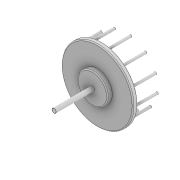
# Autodesk Inventor part: updated_base
Saved by Autodesk Inventor 2021 (Build 250183000, 183)
## iProperties
Created: 2021-06-23
Part Number: updated_base
Material: Generic
Document SubType Name: Modeling
Designer: Hp
Density: 1 g/cm^3
Appearance: Default
Mass: 195.945 g
Surface Area: 498.886 cm^2
Volume: 195.945 cm^3
Author: Hp
Autodesk Inventor part; units mm, degrees
ref_plane "YZ Plane" through (0, 0, 0) normal (1, 0, 0) x (0, 1, 0)
ref_plane "XZ Plane" through (0, 0, 0) normal (0, 1, 0) x (-1, 0, 0)
ref_plane "XY Plane" through (0, 0, 0) normal (0, 0, 1) x (1, 0, 0)
sketch "Sketch2" plane through (0, 0, 0) normal (0, 0, 1) x (1, 0, 0)
  circle A0 centre (0, 0) radius 75
  dimension "d0" = 150
  constraints: 1 centre point, 1 coincident
  measures "d0" diameter of A0
extrude "Extrusion1" add sketch "Sketch2" along normal blind 10
fillet "Fillet1" radius 2 1 edges at (-75, 0, 10)
fillet "Fillet2" radius 2 1 edges at (-75, 0, 0)
sketch "Sketch24" plane through (0, 0, 0) normal (1, 0, 0) x (0, 1, 0)
  line L0 (10, 0) -> (-10, 0) projected
  point P0 (0, 0)
sketch "Sketch25" plane through (0, 0, 0) normal (0, 0, 1) x (1, 0, 0)
  circle A0 centre (0, 0) radius 73 projected
  circle A1 centre (23.8125, -61.9125) radius 2.5
  circle A2 centre (51.5785, -41.7115) radius 2.5
  circle A3 centre (65.524, -10.334) radius 2.5
  circle A4 centre (61.9125, 23.8125) radius 2.5
  circle A5 centre (41.7115, 51.5785) radius 2.5
  circle A6 centre (10.334, 65.524) radius 2.5
  circle A7 centre (-23.8125, 61.9125) radius 2.5
  circle A8 centre (-51.5785, 41.7115) radius 2.5
  circle A9 centre (-65.524, 10.334) radius 2.5
  circle A10 centre (-61.9125, -23.8125) radius 2.5
  circle A11 centre (-41.7115, -51.5785) radius 2.5
  circle A12 centre (-10.334, -65.524) radius 2.5
  circle A13 centre (0, 0) radius 10 projected
  circle A14 centre (0, 0) radius 10 projected
  dimension "d104" = 5
  dimension "d107" = 360
  constraints: 12 centre point, 2 coincident, 25 other
  measures "d104" diameter of A1
sketch "Sketch26" plane through (0, 0, 0) normal (0, 0, -1) x (-1, 0, 0)
  point P0 (0, 0)
extrude "Extrusion6" add sketch "Sketch25" against normal blind 50 contours A2 | A3 | A4 | A5 | A6 | A7 | A8 | A9 | A10 | A11 | A12
sketch "Sketch29" plane through (0, 0, 0) normal (0, 0, 1) x (1, 0, 0)
  circle A0 centre (23.8125, -61.9125) radius 2.5
  point P0 (0, 0)
  dimension "d111" = 5
  constraints: 1 centre point
  measures "d111" diameter of A0
extrude "Extrusion7" add sketch "Sketch29" against normal blind 50
sketch "Sketch30" plane through (0, 0, 0) normal (0, 0, 1) x (1, 0, 0)
  point P0 (0, 0)
sketch "Sketch31" plane through (0, 0, 0) normal (0, 0, 1) x (1, 0, 0)
  point P0 (0, 0)
sketch "Sketch32" plane through (0, 0, 10) normal (0, 0, 1) x (1, 0, 0)
  circle A0 centre (0, 0) radius 4
  dimension "d114" = 8
  constraints: 1 centre point, 1 coincident
  measures "d114" diameter of A0
extrude "Extrusion8" cut sketch "Sketch32" against normal through all both and the other way through all
sketch "Sketch33" plane through (0, 0, 10) normal (0, 0, 1) x (1, 0, 0)
  circle A0 centre (0, 0) radius 4 projected
  circle A1 centre (0, 0) radius 31.511
  constraints: 1 centre point, 1 coincident
extrude "Extrusion9" add sketch "Sketch33" along normal blind 10
fillet "Fillet3" radius 2 1 edges at (-31.511, 0, 20)
sketch "Sketch34" plane through (0, 0, 20) normal (0, 0, 1) x (1, 0, 0)
  circle A0 centre (0, 0) radius 4 projected
  circle A1 centre (0, 0) radius 4.5
  dimension "d120" = 9
  constraints: 1 centre point, 1 coincident
  measures "d120" diameter of A1
extrude "Extrusion10" add sketch "Sketch34" along normal blind 80 contours A0 | A1
sketch "Sketch35" plane through (0, 0, 100) normal (0, 0, 1) x (1, 0, 0)
  circle A0 centre (0, 0) radius 4 projected
  circle A1 centre (0, 0) radius 4
  dimension "d123" = 8
  constraints: 1 centre point, 1 coincident
  measures "d123" diameter of A1
extrude "Extrusion11" cut sketch "Sketch35" against normal blind 10
body "Solid1"
